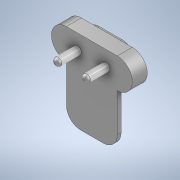
# Autodesk Inventor part: charger cover pt2
Saved by Autodesk Inventor 2022 (Build 260153000, 153)
## iProperties
Created: 2023-02-20
Part Number: charger cover pt2
Material: Iron, Malleable
Document SubType Name: Modeling
Designer: yashm
Density: 7.15 g/cm^3
Appearance: Semi-Polished
Author: yashm
Autodesk Inventor part; units mm, degrees
ref_plane "YZ Plane" through (0, 0, 0) normal (1, 0, 0) x (0, 1, 0)
ref_plane "XZ Plane" through (0, 0, 0) normal (0, 1, 0) x (-1, 0, 0)
ref_plane "XY Plane" through (0, 0, 0) normal (0, 0, 1) x (1, 0, 0)
sketch "Sketch2" plane through (0, 0, 0) normal (0, 0, 1) x (1, 0, 0)
  line L0 (0, 34.57) -> (0, 0)
  line L1 (9.5, -9.5) -> (24.5, -9.5)
  line L2 (34, 0) -> (34, 34.57)
  line L3 (9.5, 44.07) -> (24.5, 44.07)
  arc A0 (9.5, 44.07) -> (0, 34.57) centre (9.5, 34.57) ccw
  arc A1 (34, 34.57) -> (24.5, 44.07) centre (24.5, 34.57) ccw
  arc A2 (24.5, -9.5) -> (34, 0) centre (24.5, 0) ccw
  arc A3 (0, 0) -> (9.5, -9.5) centre (9.5, 0) ccw
  point P0 (0, 0)
  dimension "d5" = 9.5
  dimension "d6" = 15
  dimension "d23" = 53.57
  constraints: 8 end point, 8 point on circle, 7 tangent, 4 centre point, 2 equal radius, 2 horizontal, 2 parallel, 2 vertical, 1 coincident
  measures "d5" radius of A3
  measures "d6" distance of L3.start L3.end
  measures "d23" distance between parallel lines of L1 L3
extrude "Extrusion2" add sketch "Sketch2" along normal blind 12.5
sketch "Sketch3" plane through (0, 0, 0) normal (-1, 0, 0) x (0, 0, 1)
  line L0 (0, -9.5) -> (12.5, -9.5) projected
  line L1 (0, 23.0882) -> (10, 23.0882)
  line L2 (10, 23.0882) -> (10, -9.5)
  line L3 (10, -9.5) -> (0, -9.5)
  line L4 (0, -9.5) -> (0, 23.0882)
  line L5 (0, 34.57) -> (0, 0) projected
  dimension "d9" = 32.5882
  dimension "d10" = 10
  constraints: 8 end point, 2 parallel, 2 point on line, 1 horizontal, 1 perpendicular
  measures "d9" distance of L1.end L2.end
  measures "d10" distance between parallel lines of L4 L2
extrude "Extrusion3" cut sketch "Sketch3" against normal through all
sketch "Sketch4" plane through (0, 0, 0) normal (0, 0, -1) x (-1, 0, 0)
  line L0 (-32.5, 34.57) -> (-32.5, 23.0882)
  line L1 (0, 23.0882) -> (-34, 23.0882) projected
  line L2 (-32.5, 23.0882) -> (-1.5, 23.0882)
  line L3 (-1.5, 23.0882) -> (-1.5, 34.57)
  line L4 (-24.5, 42.57) -> (-9.5, 42.57)
  arc A0 (-1.5, 34.57) -> (-9.5, 42.57) centre (-9.5, 34.57) ccw
  arc A1 (-24.5, 42.57) -> (-32.5, 34.57) centre (-24.5, 34.57) ccw
  arc A2 (-24.5, 44.07) -> (-34, 34.57) centre (-24.5, 34.57) ccw projected
  point P0 (0, 0)
  dimension "d13" = 15
  dimension "d14" = 8
  constraints: 8 end point, 4 point on circle, 4 tangent, 2 centre point, 2 point on line, 2 vertical, 1 concentric, 1 equal radius, 1 horizontal
  measures "d13" distance of L4.start L4.end
  measures "d14" radius of A1
sketch "Sketch8" plane through (0, 0, 12.5) normal (0, 0, 1) x (1, 0, 0)
  line L0 (0, 45.57) -> (34, 45.57)
  line L1 (0, 25.5882) -> (34, 25.5882)
  line L2 (34, 0) -> (34, 34.57) projected
  line L3 (0, 34.57) -> (0, 0) projected
  line L4 (24.5, 44.07) -> (9.5, 44.07) projected
  line L5 (24.5, 44.07) -> (9.5, 44.07) projected
  arc A0 (0, 45.57) -> (0, 25.5882) centre (0, 35.5791) ccw
  arc A1 (34, 25.5882) -> (34, 45.57) centre (34, 35.5791) ccw
  point P0 (0, 23.0882)
  point P1 (17, 45.57)
  point P2 (17, 44.07)
  dimension "d25" = 1.5
  dimension "d26" = 2.5
  dimension "d40" = 0
  constraints: 4 end point, 4 point on circle, 2 centre point, 2 horizontal, 2 midpoint, 2 point on line, 2 tangent, 1 parallel
  measures "d25" distance between parallel lines of L4 L0
  measures "d26" distance from line of point (0, 23.088) L1
  measures "d40" horizontal distance of L1.start L0.start
extrude "Extrusion7" add sketch "Sketch8" against normal blind 10
extrude "Extrusion6" cut sketch "Sketch4" against normal up to surface (10 mm away)
sketch "Sketch10" plane through (0, 0, 12.5) normal (0, 0, 1) x (1, 0, 0)
  circle A0 centre (7.45, 35.5791) radius 2.52
  circle A1 centre (26.55, 35.5791) radius 2.52
  line L0 (7.45, 35.5791) -> (0, 35.5791)
  line L1 (34, 35.5791) -> (26.55, 35.5791)
  point P0 (0, 0)
  dimension "d29" = 19.1
  dimension "d30" = 5.04
  dimension "d31" = 0
  dimension "d32" = 0
  constraints: 4 end point, 2 centre point, 1 collinear, 1 equal radius
  measures "d29" distance of L1.end L0.start
  measures "d30" diameter of A0
  measures "d31" vertical distance of L0.end L0.start
  measures "d32" vertical distance of L1.start L1.end
extrude "Extrusion8" cut sketch "Sketch10" against normal blind 10
sketch "Sketch11" plane through (0, 0, 12.5) normal (0, 0, 1) x (1, 0, 0)
  circle A0 centre (7.45, 35.5791) radius 2.52 projected
  circle A1 centre (26.55, 35.5791) radius 2.52 projected
  point P0 (0, 0)
extrude "Extrusion9" add sketch "Sketch11" along normal blind 15
fillet "Fillet1" radius 2 2 edges at (4.93, 35.5791, 27.5) (24.03, 35.5791, 27.5)
body "Solid2"
